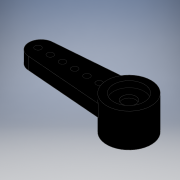
# Autodesk Inventor part: TP-MG92B_HAT
Saved by Autodesk Inventor 2017 (Build 210142000, 142)
## iProperties
Created: 2017-09-24
Part Number: TP-MG92B_HAT
Material: Generic
Document SubType Name: Modeling
Designer: Alexander Miller
Density: 1 g/cm^3
Appearance: Default
servo_hat_A: 7,250 mm
Author: Alexander Miller
Autodesk Inventor part; units mm, degrees
ref_plane "YZ Plane" through (0, 0, 0) normal (1, 0, 0) x (0, 1, 0)
ref_plane "XZ Plane" through (0, 0, 0) normal (0, 1, 0) x (-1, 0, 0)
ref_plane "XY Plane" through (0, 0, 0) normal (0, 0, 1) x (1, 0, 0)
sketch "Sketch1" plane through (0, 0, 0) normal (0, 1, 0) x (-1, 0, 0)
  line L0 (0, 3.625) -> (0, -16.375) construction
  circle A0 centre (0, 0) radius 3.625
  circle A1 centre (0, -14.375) radius 2 construction
  line L1 (3, -2.0349) -> (-3, -2.0349)
  line L2 (3, -2.0349) -> (2, -14.375)
  line L3 (-3, -2.0349) -> (-2, -14.375)
  arc A2 (-2, -14.375) -> (2, -14.375) centre (0, -14.375) ccw
  point P0 (0, -2.0349)
  dimension "d0" = 20
  dimension "d1" = 7.25
  dimension "d2" = 4
  dimension "d3" = 6
  constraints: 8 end point, 7 point on circle, 3 centre point, 2 horizontal alignment, 2 point on line, 1 coincident, 1 concentric, 1 horizontal, 1 midpoint, 1 vertical, 1 vertical alignment
  measures "d0" distance of L0.start L0.end
  measures "d1" diameter of A0
  measures "d2" diameter of A1
  measures "d3" distance of L1.start L1.end
extrude "Extrusion1" add sketch "Sketch1" along normal blind 2
sketch "Sketch2" plane through (0, 2, 0) normal (0, 1, 0) x (1, 0, 0)
  circle A0 centre (0, 0) radius 3.625
  arc A1 (-3, 2.0349) -> (3, 2.0349) centre (0, 0) ccw projected
  constraints: 2 concentric, 1 centre point
extrude "Extrusion2" add sketch "Sketch2" along normal blind 1
sketch "Sketch3" plane through (0, 0, 0) normal (0, -1, 0) x (1, 0, 0)
  circle A0 centre (0, 0) radius 3.625
  arc A1 (3, -2.0349) -> (-3, -2.0349) centre (0, 0) ccw projected
  constraints: 2 concentric, 1 centre point
extrude "Extrusion3" add sketch "Sketch3" along normal blind 2.5
sketch "Sketch4" plane through (0, 3, 0) normal (0, 1, 0) x (1, 0, 0)
  circle A0 centre (0, 0) radius 2.5
  circle A1 centre (0, 0) radius 3.625 projected
  dimension "d10" = 5
  constraints: 1 centre point, 1 concentric
  measures "d10" diameter of A0
extrude "Extrusion4" cut sketch "Sketch4" against normal blind 1 contours A0
sketch "Sketch5" plane through (0, -2.5, 0) normal (0, -1, 0) x (1, 0, 0)
  circle A0 centre (0, 0) radius 2.5
  circle A1 centre (0, 0) radius 3.625 projected
  dimension "d13" = 5
  constraints: 1 centre point, 1 concentric
  measures "d13" diameter of A0
extrude "Extrusion5" cut sketch "Sketch5" against normal blind 4 contours A0
sketch "Sketch6" plane through (0, 2, 0) normal (0, 1, 0) x (1, 0, 0)
  circle A0 centre (0, 0) radius 1.125
  circle A1 centre (0, 0) radius 2.5 projected
  dimension "d16" = 2.25
  constraints: 1 centre point, 1 concentric
  measures "d16" diameter of A0
extrude "Extrusion6" cut sketch "Sketch6" against normal through all contours A0
sketch "Sketch7" plane through (0, 2, 0) normal (0, 1, 0) x (1, 0, 0)
  circle A0 centre (0, 4.875) radius 0.5
  circle A1 centre (0, 6.875) radius 0.5
  circle A2 centre (0, 8.875) radius 0.5
  circle A3 centre (0, 10.875) radius 0.5
  circle A4 centre (0, 12.875) radius 0.5
  circle A5 centre (0, 14.875) radius 0.5
  arc A6 (2, 14.375) -> (-2, 14.375) centre (0, 14.375) ccw projected
  point P0 (0, 0)
  point P1 (0, 16.375)
  dimension "d19" = 1
  dimension "d20" = 2
  dimension "d21" = 2
  dimension "d22" = 2
  dimension "d23" = 2
  dimension "d24" = 2
  dimension "d25" = 1.5
  constraints: 7 vertical alignment, 6 centre point, 5 equal radius, 1 point on circle
  measures "d19" diameter of A0
  measures "d20" distance of A4.centre A5.centre
  measures "d21" distance of A3.centre A4.centre
  measures "d22" distance of A2.centre A3.centre
  measures "d23" distance of A1.centre A2.centre
  measures "d24" distance of A0.centre A1.centre
  measures "d25" distance of A5.centre point (0, 16.375)
extrude "Extrusion7" cut sketch "Sketch7" against normal through all
equation "\"d1\" = servo_hat_A"
equation "\"servo_hat_A\" = 7.25"
body "Solid1"
